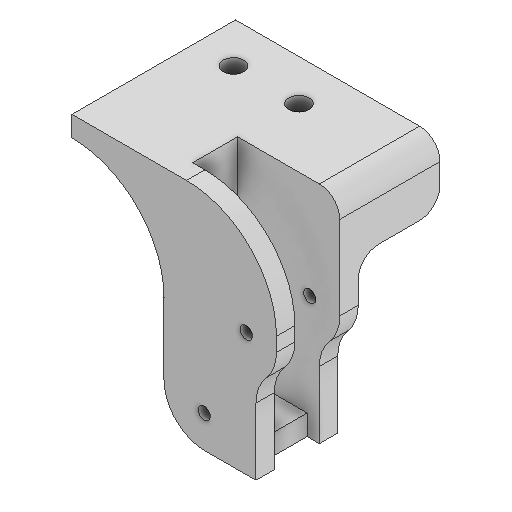
# Autodesk Inventor part: SOPORTE_FDC
Saved by Autodesk Inventor 2024 (Build 280153000, 153)
## iProperties
Created: 2024-08-21
Part Number: SOPORTE_FDC
Material: Generic
Document SubType Name: Modeling
Designer: Jhuliams
Density: 1 g/cm^3
Appearance: Default
Author: Jhuliams
Autodesk Inventor part; units mm, degrees
ref_plane "YZ Plane" through (0, 0, 0) normal (1, 0, 0) x (0, 1, 0)
ref_plane "XZ Plane" through (0, 0, 0) normal (0, 1, 0) x (-1, 0, 0)
ref_plane "XY Plane" through (0, 0, 0) normal (0, 0, 1) x (1, 0, 0)
sketch "Sketch1" plane through (0, 0, 0) normal (0, 1, 0) x (-1, 0, 0)
  line L0 (22.5, 10) -> (-22.5, 10)
  line L1 (-22.5, 10) -> (-22.5, -10)
  line L2 (-22.5, -10) -> (22.5, -10)
  line L3 (22.5, -10) -> (22.5, 10)
  line L4 (22.5, 10) -> (-22.5, -10) construction
  line L5 (-22.5, 10) -> (22.5, -10) construction
  point P0 (0, 0)
  dimension "d0" = 45
  dimension "d1" = 20
  constraints: 12 end point, 2 midpoint, 2 parallel, 1 horizontal, 1 perpendicular
  measures "d0" distance of L2.end L1.end
  measures "d1" distance of L1.end L0.end
extrude "Extrusion1" add sketch "Sketch1" along normal blind 5
sketch "Sketch2" plane through (0, 0, 0) normal (0, -1, 0) x (1, 0, 0)
  line L0 (22.5, 10) -> (22.5, -10) projected
  line L1 (22.5, 10) -> (0, 10)
  line L2 (0, 10) -> (0, 5)
  line L3 (0, 5) -> (22.5, 5)
  line L4 (22.5, 5) -> (22.5, 10)
  point P0 (0, 0)
  dimension "d4" = 22.5
  dimension "d5" = 5
  constraints: 8 end point, 2 parallel, 1 horizontal, 1 perpendicular
  measures "d4" distance of L3.end L2.end
  measures "d5" distance of L2.end L1.end
extrude "Extrusion2" add sketch "Sketch2" along normal blind 50
fillet "Fillet1" radius 22.5 1 edges at (0, 0, 7.5)
sketch "Sketch3" plane through (-22.5, 5, 10) normal (0, 0, 1) x (1, 0, 0)
  arc A0 (22.5, -27.5) -> (0, -5) centre (0, -27.5) ccw projected
  line L0 (22.5, -27.5) -> (22.5, -55) projected
  line L1 (45, -55) -> (22.5, -55) projected
  line L2 (45, 0) -> (45, -55) projected
  line L3 (0, 0) -> (45, 0) projected
  line L4 (0, -5) -> (0, 0) projected
  point P0 (22.5, -5)
extrude "Extrusion3" add sketch "Sketch3" along normal blind 15
sketch "Sketch7" plane through (0, 5, 0) normal (0, 1, 0) x (1, 0, 0)
  line L0 (22.5, -5) -> (-22.5, -5) projected
  line L1 (22.5, 10) -> (22.5, -25) projected
  line L2 (22.5, -5) -> (22.5, -25)
  line L3 (42.5, -20.5) -> (2.5, -20.5)
  line L4 (2.5, -20.5) -> (2.5, -9.5)
  line L5 (2.5, -9.5) -> (42.5, -9.5)
  line L6 (42.5, -9.5) -> (42.5, -20.5)
  line L7 (42.5, -20.5) -> (2.5, -9.5) construction
  line L8 (2.5, -20.5) -> (42.5, -9.5) construction
  point P0 (0, 0)
  point P1 (22.5, -15)
  dimension "d16" = 40
  dimension "d17" = 11
  constraints: 14 end point, 3 midpoint, 2 parallel, 1 collinear, 1 horizontal, 1 perpendicular
  measures "d16" distance of L4.end L5.end
  measures "d17" distance of L3.end L4.end
extrude "Extrusion5" cut sketch "Sketch7" against normal blind 50
sketch "Sketch8" plane through (0, -45, 0) normal (0, 1, 0) x (1, 0, 0)
  line L0 (22.5, -5) -> (22.5, -25) projected
  line L1 (22.5, -15) -> (7.5, -15)
  line L2 (22.5, -15) -> (37.5, -15) construction
  line L3 (2.5, -20.5) -> (12.5, -20.5)
  line L4 (12.5, -20.5) -> (12.5, -9.5)
  line L5 (12.5, -9.5) -> (2.5, -9.5)
  line L6 (2.5, -9.5) -> (2.5, -20.5)
  line L7 (2.5, -20.5) -> (12.5, -9.5) construction
  line L8 (12.5, -20.5) -> (2.5, -9.5) construction
  line L9 (7.5, -20.5) -> (7.5, -9.5)
  point P0 (0, 0)
  dimension "d20" = 15
  dimension "d21" = 180
  dimension "d22" = 10
  dimension "d23" = 11
  constraints: 18 end point, 5 midpoint, 2 horizontal, 2 parallel, 2 perpendicular, 1 collinear
  measures "d20" distance of L1.start L1.end
  measures "d21" angle of L1 L2
  measures "d22" distance of L5.end L4.end
  measures "d23" distance of L4.end L3.end
extrude "Extrusion6" add sketch "Sketch8" along normal blind 15 contours L9 L3 L6 L5
sketch "Sketch9" plane through (0, -45, 0) normal (0, 1, 0) x (1, 0, 0)
  line L0 (7.5, -9.5) -> (22.5, -9.5) projected
  line L1 (22.5, -9.5) -> (19.5, -9.5)
  line L2 (19.5, -9.5) -> (19.5, -20.5)
  line L3 (19.5, -20.5) -> (22.5, -20.5)
  line L4 (22.5, -20.5) -> (22.5, -9.5)
  point P0 (0, 0)
  dimension "d26" = 3
  dimension "d27" = 11
  constraints: 8 end point, 2 parallel, 1 horizontal, 1 perpendicular
  measures "d26" distance of L3.end L2.end
  measures "d27" distance of L2.end L1.end
extrude "Extrusion7" cut sketch "Sketch9" against normal blind 15
fillet "Fillet2" radius 10 1 edges at (0, -50, 15)
sketch "Sketch10" plane through (-22.5, 5, 25) normal (0, 0, 1) x (1, 0, 0)
  circle A0 centre (32.35, -47.1) radius 1.5 projected
  circle A1 centre (42.65, -24.9) radius 1.5 projected
  point P0 (22.5, -5)
extrude "Extrusion8" cut sketch "Sketch10" against normal blind 20
sketch "Sketch11" plane through (22.5, 0, -10) normal (1, 0, 0) x (0, 0, -1)
  line L0 (-19.5, 5) -> (-19.5, -50) projected
  line L1 (-15, -50) -> (-19.5, -50) projected
  line L2 (-15, 0) -> (-15, -50) projected
  line L3 (-15, 0) -> (0, 0) projected
  line L4 (0, 0) -> (0, 5) projected
  line L5 (0, 5) -> (-19.5, 5) projected
  line L6 (-30.5, -50) -> (-30.5, 5) projected
  line L7 (-30.5, 5) -> (-35, 5) projected
  line L8 (-35, -50) -> (-35, 5) projected
  line L9 (-30.5, -50) -> (-35, -50) projected
  point P0 (-10, 0)
extrude "Extrusion9" add sketch "Sketch11" along normal blind 5
sketch "Sketch12" plane through (0, -50, 0) normal (0, -1, 0) x (1, 0, 0)
  line L0 (10, 5) -> (27.5, 5) projected
  line L1 (27.5, 5) -> (22.5, 5)
  line L2 (22.5, 5) -> (22.5, 25)
  line L3 (22.5, 25) -> (27.5, 25)
  line L4 (27.5, 25) -> (27.5, 5)
  point P0 (0, 0)
  dimension "d35" = 5
  dimension "d36" = 20
  constraints: 8 end point, 2 parallel, 1 horizontal, 1 perpendicular
  measures "d35" distance of L2.end L3.end
  measures "d36" distance of L1.end L2.end
extrude "Extrusion10" cut sketch "Sketch12" against normal blind 25
fillet "Fillet3" radius 10 4 edges at (27.5, -25, 7.25) (22.5, -25, 7.25) (27.5, -25, 22.75) (22.5, -25, 22.75)
sketch "Sketch13" plane through (0, 0, 0) normal (0, -1, 0) x (1, 0, 0)
  line L0 (27.5, -10) -> (17.5, -10)
  line L1 (17.5, -10) -> (17.5, 5)
  line L2 (17.5, 5) -> (27.5, 5)
  line L3 (27.5, 5) -> (27.5, -10)
  point P0 (0, 0)
  dimension "d40" = 10
  dimension "d41" = 15
  constraints: 8 end point, 2 parallel, 1 horizontal, 1 perpendicular
  measures "d40" distance of L1.end L2.end
  measures "d41" distance of L0.end L1.end
extrude "Extrusion11" add sketch "Sketch13" along normal blind 10
sketch "Sketch14" plane through (0, 5, 0) normal (0, 1, 0) x (1, 0, 0)
  line L0 (-22.5, 10) -> (27.5, 10) projected
  line L1 (-22.5, 10) -> (-13, 10)
  line L2 (-13, 10) -> (-13, 5)
  line L3 (-13, 5) -> (3, 5)
  circle A0 centre (-13, 5) radius 2.5
  circle A1 centre (3, 5) radius 2.5
  point P0 (0, 0)
  dimension "d45" = 9.5
  dimension "d46" = 5
  dimension "d47" = 16
  dimension "d48" = 90
  dimension "d49" = 5
  dimension "d50" = 5
  constraints: 6 end point, 2 centre point, 2 coincident, 2 perpendicular, 1 point on line
  measures "d45" distance of L0.start L1.end
  measures "d46" distance of L1.end L2.end
  measures "d47" distance of L2.end L3.end
  measures "d48" angle of L3 L2
  measures "d49" diameter of A0
  measures "d50" diameter of A1
extrude "Extrusion12" cut sketch "Sketch14" against normal blind 10
sketch "Sketch15" plane through (-22.5, 0, -10) normal (0, 0, -1) x (-1, 0, 0)
  line L0 (0, 0) -> (-40, 0) projected
  line L1 (0, 0) -> (0, 5) projected
  line L2 (0, 5) -> (-50, 5) projected
  line L3 (-50, 5) -> (-50, -10) projected
  line L4 (-40, -10) -> (-50, -10) projected
  line L5 (-40, 0) -> (-40, -10) projected
  point P0 (-22.5, 0)
extrude "Extrusion13" add sketch "Sketch15" along normal blind 5
fillet "Fillet5" radius 5 1 edges at (-2.5, 0, -15)
fillet "Fillet6" radius 5 2 edges at (22.5, -10, 5) (22.5, -10, -15)
fillet "Fillet7" radius 22 1 edges at (27.5, 5, 22.75)
fillet "Fillet8" radius 5 1 edges at (27.5, 5, -2.75)
body "Solid1"
